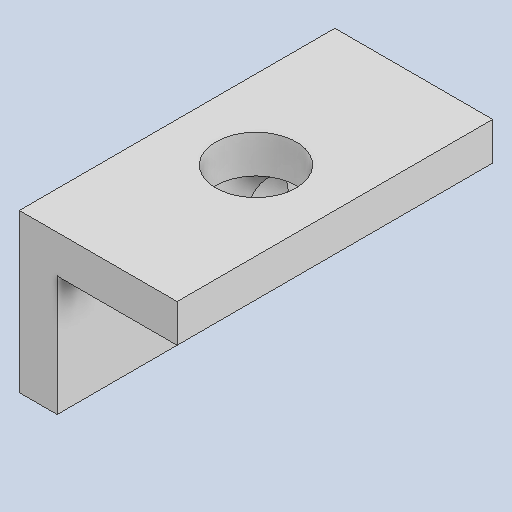
# Autodesk Inventor part: Roter_shaft_support_top
Saved by Autodesk Inventor 2026.1 (Build 301233000, 233)
## iProperties
Created: 2025-09-10
Part Number: Roter_shaft_support_top
Material: Generic
Document SubType Name: Modeling
Designer: sraav
Density: 1 g/cm^3
Appearance: Default
Author: sraav
Autodesk Inventor part; units mm, degrees
ref_plane "YZ Plane" through (0, 0, 0) normal (1, 0, 0) x (0, 1, 0)
ref_plane "XZ Plane" through (0, 0, 0) normal (0, 1, 0) x (-1, 0, 0)
ref_plane "XY Plane" through (0, 0, 0) normal (0, 0, 1) x (1, 0, 0)
sketch "Sketch1" plane through (0, 0, 0) normal (0, 1, 0) x (-1, 0, 0)
  line L0 (0, 0) -> (0, 50)
  line L1 (0, 50) -> (-25, 50)
  line L2 (-25, 50) -> (-25, 0)
  line L3 (-25, 0) -> (0, 0)
  circle A0 centre (-12.5, 25) radius 6.35
  dimension "d0" = 50
  dimension "d1" = 25
  dimension "d2" = 12.7
  constraints: 8 end point, 2 perpendicular, 1 centre point, 1 horizontal, 1 vertical
  measures "d0" distance of L0.start L0.end
  measures "d1" distance of L0.end L1.end
  measures "d2" diameter of A0
extrude "Extrusion1" add sketch "Sketch1" against normal blind 6
sketch "Sketch2" plane through (0, -6, 0) normal (0, -1, 0) x (1, 0, 0)
  line L0 (0, 50) -> (0, 0) projected
  line L1 (0, 50) -> (6, 50)
  line L2 (25, 50) -> (0, 50) projected
  line L3 (6, 50) -> (6, 0)
  line L4 (0, 0) -> (25, 0) projected
  line L5 (6, 0) -> (0, 0)
  line L6 (0, 0) -> (0, 50)
  dimension "d5" = 6
  constraints: 8 end point, 2 collinear, 1 perpendicular, 1 point on line
  measures "d5" distance of L0.start L1.end
extrude "Extrusion2" add sketch "Sketch2" along normal blind 19
sketch "Sketch3" plane through (6, -6, 50) normal (1, 0, 0) x (0, 0, -1)
  circle A0 centre (16.6667, -6.5) radius 3.25
  circle A1 centre (33.3333, -6.5) radius 3.25
  point P0 (50, 6)
  dimension "d8" = 6.5
  dimension "d9" = 6.5
  constraints: 2 centre point
  measures "d8" diameter of A0
  measures "d9" diameter of A1
hole "Hole1" at (6, -12.5, 33.3333) at (6, -12.5, 16.6667) direction (-1, 0, 0) diameter 6.5 depth 111
body "Solid1"
